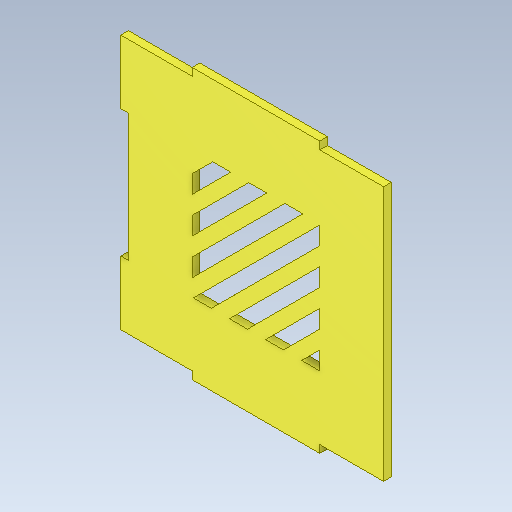
# Autodesk Inventor part: Control lateral
Saved by Autodesk Inventor 2020 (Build 240168000, 168)
## iProperties
Created: 2020-03-09
Part Number: Control lateral
Material: Genérico
Document SubType Name: Modeling
Designer: joser
Density: 1 g/cm^3
Appearance: Suave - Amarillo
Author: joser
Autodesk Inventor part; units mm, degrees
ref_plane "YZ Plane" through (0, 0, 0) normal (1, 0, 0) x (0, 1, 0)
ref_plane "XZ Plane" through (0, 0, 0) normal (0, 1, 0) x (-1, 0, 0)
ref_plane "XY Plane" through (0, 0, 0) normal (0, 0, 1) x (1, 0, 0)
sketch "Boceto1" plane through (0, 0, 0) normal (0, 0, 1) x (1, 0, 0)
  line L0 (0, 100) -> (0, 0)
  line L1 (-100, 25) -> (-100, 75)
  line L2 (-75, 0) -> (-75, -3)
  line L3 (-75, -3) -> (-25, -3)
  line L4 (-25, -3) -> (-25, 0)
  line L5 (0, 0) -> (-25, 0)
  line L6 (-103, 100) -> (-103, 75)
  line L7 (-103, 75) -> (-100, 75)
  line L8 (-103, 0) -> (-103, 25)
  line L9 (-103, 25) -> (-100, 25)
  line L10 (-103, 0) -> (-75, 0)
  line L11 (-75, 100) -> (-75, 103)
  line L12 (-75, 103) -> (-25, 103)
  line L13 (-25, 103) -> (-25, 100)
  line L14 (0, 100) -> (-25, 100)
  line L15 (-75, 100) -> (-103, 100)
  line L16 (-75, 66.9731) -> (-66.9731, 75)
  line L17 (-75, 66.9731) -> (-63.6482, 66.9731) construction
  line L18 (-75, 59.902) -> (-59.902, 75)
  line L19 (-75, 52.8309) -> (-52.8309, 75)
  line L20 (-75, 45.7599) -> (-45.7599, 75)
  line L21 (-75, 38.6888) -> (-38.6888, 75)
  line L22 (-75, 31.6177) -> (-31.6177, 75)
  line L23 (-74.5467, 25) -> (-25, 74.5467)
  line L24 (-67.4756, 25) -> (-25, 67.4756)
  line L25 (-60.4045, 25) -> (-25, 60.4045)
  line L26 (-53.3335, 25) -> (-25, 53.3335)
  line L27 (-46.2624, 25) -> (-25, 46.2624)
  line L28 (-39.1913, 25) -> (-25, 39.1913)
  line L29 (-32.1203, 25) -> (-25, 32.1203)
  line L30 (-66.9731, 75) -> (-59.902, 75)
  line L31 (-75, 59.902) -> (-75, 66.9731)
  line L32 (-75, 31.6177) -> (-75, 38.6888)
  line L33 (-75, 45.7599) -> (-75, 52.8309)
  line L34 (-52.8309, 75) -> (-45.7599, 75)
  line L35 (-38.6888, 75) -> (-31.6177, 75)
  line L36 (-67.4756, 25) -> (-74.5467, 25)
  line L37 (-25, 74.5467) -> (-25, 67.4756)
  line L38 (-25, 60.4045) -> (-25, 53.3335)
  line L39 (-53.3335, 25) -> (-60.4045, 25)
  line L40 (-25, 25) -> (-32.1203, 25)
  line L41 (-39.1913, 25) -> (-46.2624, 25)
  line L42 (-25, 46.2624) -> (-25, 39.1913)
  line L43 (-25, 32.1203) -> (-25, 25)
  dimension "d1" = 100
  dimension "d4" = 50
  dimension "d5" = 25
  dimension "d7" = 25
  dimension "d8" = 25
  dimension "d9" = 3
  dimension "d10" = 3
  dimension "d11" = 100
  dimension "d13" = 50
  dimension "d14" = 3
  dimension "d15" = 45
  dimension "d16" = 5
  dimension "d17" = 5
  dimension "d18" = 5
  dimension "d19" = 5
  dimension "d20" = 5
  dimension "d21" = 5
  dimension "d22" = 5
  dimension "d25" = 5
  dimension "d26" = 5
  dimension "d27" = 5
  dimension "d28" = 5
  dimension "d29" = 5
  dimension "d30" = 25
  dimension "d31" = 25
  dimension "d32" = 11.3518
  constraints: 88 end point, 35 parallel, 21 perpendicular, 16 collinear, 7 horizontal, 2 vertical, 1 coincident, 1 equal length
  measures "d1" distance of L0.start L0.end
  measures "d4" distance of L2.end L3.end
  measures "d5" distance between parallel lines of L0 L4
  measures "d7" distance of L6.start L6.end
  measures "d8" distance of L8.start L8.end
  measures "d9" distance between parallel lines of L1 L6
  measures "d10" distance between parallel lines of L10 L3
  measures "d11" distance between parallel lines of L0 L1
  measures "d13" distance of L11.end L12.end
  measures "d14" distance between parallel lines of L15 L12
  measures "d15" angle of L17 L16
  measures "d16" distance between parallel lines of L18 L16
  measures "d17" distance between parallel lines of L19 L18
  measures "d18" distance between parallel lines of L19 L20
  measures "d19" distance between parallel lines of L20 L21
  measures "d20" distance between parallel lines of L21 L22
  measures "d21" distance between parallel lines of L22 L23
  measures "d22" distance between parallel lines of L23 L24
  measures "d25" distance between parallel lines of L24 L25
  measures "d26" distance between parallel lines of L25 L26
  measures "d27" distance between parallel lines of L26 L27
  measures "d28" distance between parallel lines of L27 L28
  measures "d29" distance between parallel lines of L28 L29
  measures "d30" distance between parallel lines of L0 L43
  measures "d31" distance between parallel lines of L5 L41
  measures "d32" distance of L16.start L16.end
extrude "Extrusión1" add sketch "Boceto1" along normal blind 3
